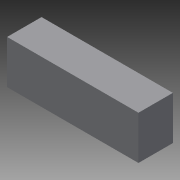
# Autodesk Inventor part: lipo4s
Saved by Autodesk Inventor 2014 SP1 (Build 180222100, 222)
## iProperties
Created: 2015-08-03
Part Number: lipo4s
Material: Générique
Document SubType Name: Modeling
Designer: astralien3000
Density: 1 g/cm^3
Appearance: Par défaut
Author: astralien3000
Autodesk Inventor part; units mm, degrees
ref_plane "YZ Plane" through (0, 0, 0) normal (1, 0, 0) x (0, 1, 0)
ref_plane "XZ Plane" through (0, 0, 0) normal (0, 1, 0) x (-1, 0, 0)
ref_plane "XY Plane" through (0, 0, 0) normal (0, 0, 1) x (1, 0, 0)
sketch "Esquisse1" plane through (0, 0, 0) normal (0, 1, 0) x (-1, 0, 0)
  line L0 (-72.5, 24) -> (72.5, 24)
  line L1 (72.5, 24) -> (72.5, -24)
  line L2 (72.5, -24) -> (-72.5, -24)
  line L3 (-72.5, -24) -> (-72.5, 24)
  point P0 (0, 0)
  dimension "d0" = 48
  dimension "d1" = 145
  dimension "d2" = 72.5
  dimension "d3" = 24
  constraints: 8 end point, 2 parallel, 1 horizontal, 1 perpendicular
  measures "d0" distance between parallel lines of L2 L0
  measures "d1" distance of L0.start L0.end
  measures "d2" distance from line of L1 point (0, 0)
  measures "d3" distance from line of point (0, 0) L0
extrude "Extrusion1" add sketch "Esquisse1" along normal blind 38
equation "\"d2\" = 0.5 * d1"
equation "\"d3\" = 0.5 * d0"
